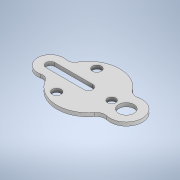
# Autodesk Inventor part: Part11
Saved by Autodesk Inventor 2021 (Build 250183000, 183)
## iProperties
Created: 2022-04-24
Part Number: Part11
Material: Generic
Document SubType Name: Modeling
Designer: hp
Density: 1 g/cm^3
Appearance: Default
Author: hp
Autodesk Inventor part; units mm, degrees
ref_plane "YZ Plane" through (0, 0, 0) normal (1, 0, 0) x (0, 1, 0)
ref_plane "XZ Plane" through (0, 0, 0) normal (0, 1, 0) x (-1, 0, 0)
ref_plane "XY Plane" through (0, 0, 0) normal (0, 0, 1) x (1, 0, 0)
sketch "Sketch1" plane through (0, 0, 0) normal (0, 1, 0) x (-1, 0, 0)
  arc A0 (97.7884, -35.051) -> (97.7884, 35.051) centre (106, 0) ccw
  arc A1 (75.9623, 44.4267) -> (97.7884, 35.051) centre (93.2264, 54.5237) ccw
  arc A2 (97.7884, -35.051) -> (75.9623, -44.4267) centre (93.2264, -54.5237) ccw
  arc A3 (-95.7901, 43.8265) -> (-95.7901, -43.8265) centre (-106, 0) ccw
  arc A4 (-95.7901, 43.8265) -> (-70.1803, 53.0916) centre (-90.1179, 68.1745) ccw
  arc A5 (-70.1803, -53.0916) -> (-95.7901, -43.8265) centre (-90.1179, -68.1745) ccw
  arc A6 (75.9623, 44.4267) -> (-70.1803, 53.0916) centre (0, 0) ccw
  arc A7 (-70.1803, -53.0916) -> (75.9623, -44.4267) centre (0, 0) ccw
  circle A8 centre (0, 0) radius 65
  circle A9 centre (-65, 0) radius 11.5
  circle A10 centre (-106, 0) radius 21.5
  arc A11 (0, 12.5) -> (0, -12.5) centre (0, 0) ccw
  arc A12 (106, -12.5) -> (106, 12.5) centre (106, 0) ccw
  line L0 (106, 12.5) -> (0, 12.5)
  line L1 (0, -12.5) -> (106, -12.5)
  line L2 (0, 0) -> (32.5, -56.2917)
  line L3 (-12.5, 0) -> (-53.5, 0)
  line L4 (0, 0) -> (23.2902, 40.3398)
  line L5 (23.2902, 40.3398) -> (32.5, 56.2917)
  circle A13 centre (32.5, 56.2917) radius 12.5
  circle A14 centre (32.5, -56.2917) radius 12.5
  dimension "d13" = 23
  dimension "d1" = 72
  dimension "d2" = 106
  dimension "d3" = 40
  dimension "d4" = 0
  dimension "d5" = 40
  dimension "d7" = 90
  dimension "d8" = 212
  dimension "d9" = 50
  dimension "d10" = 50
  dimension "d11" = 0
  dimension "d12" = 130
  dimension "d14" = 43
  dimension "d15" = 25
  dimension "d16" = 25
  dimension "d18" = 120
  dimension "d19" = 120
  dimension "d20" = 25
  dimension "d21" = 25
  constraints: 24 point on circle, 14 centre point, 12 end point, 7 coincident, 5 tangent, 1 horizontal, 1 horizontal alignment, 1 parallel, 2 other
  measures "d1" diameter of A0
  measures "d2" distance of point (0, 0) A0.centre
  measures "d3" diameter of A1
  measures "d4" vertical distance of point (0, 0) A0.centre
  measures "d5" diameter of A2
  measures "d7" diameter of A3
  measures "d8" distance of A0.centre A3.centre
  measures "d9" diameter of A4
  measures "d10" diameter of A5
  measures "d11" vertical distance of point (0, 0) A3.centre
  measures "d12" diameter of A8
  measures "d14" diameter of A10
  measures "d15" diameter of A11
  measures "d16" diameter of A12
  measures "d18" angle of L3 L2
  measures "d19" angle of L3 L4
  measures "d20" diameter of A13
  measures "d21" diameter of A14
extrude "Extrusion1" add sketch "Sketch1" along normal blind 10 contours A2 A7 A5 A3 A4 A6 A1 A0 | L0 L4 L5 A13 A8 | A8 A14 L2 L1 | L0 A11 L3 A9 A8 A13 L5 L4 | L2 A14 A8 A9 L3 A11 L1
equation "\"d5\" = d3"
equation "\"d10\" = d9"
body "Solid1"
